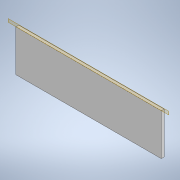
# Autodesk Inventor part: wooden_backcover
Saved by Autodesk Inventor 2020 (Build 240168000, 168)
## iProperties
Created: 2019-07-26
Part Number: wooden_backcover
Material: Generic
Document SubType Name: Modeling
Designer: erwin
Density: 1 g/cm^3
Appearance: Default
Author: erwin
Autodesk Inventor part; units mm, degrees
ref_plane "YZ Plane" through (0, 0, 0) normal (1, 0, 0) x (0, 1, 0)
ref_plane "XZ Plane" through (0, 0, 0) normal (0, 1, 0) x (-1, 0, 0)
ref_plane "XY Plane" through (0, 0, 0) normal (0, 0, 1) x (1, 0, 0)
ref_plane "Work Plane1" through (0, 0, 0) normal (0, 0, 1) x (1, 0, 0)
sketch "Sketch1" plane through (0, 0, 0) normal (0, 0, 1) x (1, 0, 0)
  line L0 (612, -44.7721) -> (612, -100.7605) projected
  line L1 (0, 0) -> (612, 0) projected
  line L2 (612, -176) -> (0, -176) projected
  line L3 (612, 0) -> (0, 0)
  line L4 (0, 0) -> (0, -176)
  line L5 (0, -176) -> (612, -176)
  line L6 (612, -176) -> (612, 0)
  constraints: 8 end point, 2 parallel, 1 horizontal, 1 perpendicular
extrude "Extrusion1" add sketch "Sketch1" against normal blind 12
thicken "Thicken1" operation add thickness 1 both sides no extend neighbours yes toward (1, 0, 0) faces at (0, -58.6667, -4) (204, -176, -4) (612, -29.8481, -4) (612, -82.0977, -4) (612, -150.9202, -4) (408, 0, -4)
body "Solid1"
